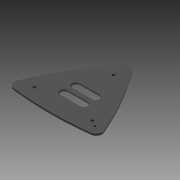
# Autodesk Inventor part: TOP PLATE
Saved by Autodesk Inventor 2013 (Build 170138000, 138)
## iProperties
Created: 2013-12-04
Part Number: TOP PLATE
Material: Generic
Document SubType Name: Modeling
Designer: employee
Density: 1 g/cm^3
Author: employee
Autodesk Inventor part; units mm, degrees
ref_plane "YZ Plane" through (0, 0, 0) normal (1, 0, 0) x (0, 1, 0)
ref_plane "XZ Plane" through (0, 0, 0) normal (0, 1, 0) x (-1, 0, 0)
ref_plane "XY Plane" through (0, 0, 0) normal (0, 0, 1) x (1, 0, 0)
sketch "Sketch1" plane through (0, 0, 0) normal (0, 0, 1) x (1, 0, 0)
  line L0 (0, -144.337567) -> (-125, 72.168784) construction
  line L1 (-125, 72.168784) -> (125, 72.168784) construction
  line L2 (125, 72.168784) -> (0, -144.337567) construction
  line L3 (0, 173.205081) -> (150, -86.60254) construction
  line L4 (150, -86.60254) -> (-150, -86.60254) construction
  line L5 (-150, -86.60254) -> (0, 173.205081) construction
  circle A0 centre (-150, -86.60254) radius 1.5875
  circle A1 centre (150, -86.60254) radius 1.5875
  circle A2 centre (0, 173.205081) radius 1.5875
  circle A3 centre (-125, 72.168784) radius 4.25
  circle A4 centre (125, 72.168784) radius 4.25
  circle A5 centre (0, -144.337567) radius 4.25
  circle A6 centre (-150, -86.60254) radius 25 construction
  line L6 (-250.015109, -144.34629) -> (0, 288.692581) construction
  line L7 (0, 288.692581) -> (250.015109, -144.34629) construction
  line L8 (250.015109, -144.34629) -> (-250.015109, -144.34629) construction
  arc A7 (-225.583531, -102.508939) -> (-201.567111, -144.106599) centre (-197.772126, -114.18379) ccw
  circle A8 centre (-125, 72.168784) radius 12.5 construction
  arc A9 (24.01642, 246.615539) -> (-24.01642, 246.615539) centre (0, 228.367581) ccw
  arc A10 (201.567111, -144.106599) -> (225.583531, -102.508939) centre (197.772126, -114.18379) ccw
  arc A11 (-24.01642, 246.615539) -> (-225.583531, -102.508939) centre (1251.593518, -722.607855) ccw
  arc A12 (225.583531, -102.508939) -> (24.01642, 246.615539) centre (-1251.593518, -722.607855) ccw
  arc A13 (-201.567111, -144.106599) -> (201.567111, -144.106599) centre (0, 1445.215709) ccw
  circle A14 centre (0, 228.367581) radius 1.5875
  circle A15 centre (-197.772126, -114.18379) radius 1.5875
  circle A16 centre (197.772126, -114.18379) radius 1.5875
  point P0 (0, 0)
  point P1 (0, 0)
  point P2 (0, 0)
  point P3 (0, 0)
  dimension "d0" = 300
  dimension "d1" = 250
  dimension "d2" = 3.175
  dimension "d3" = 8.5
  dimension "d4" = 50
  dimension "d5" = 60.325
  dimension "d6" = 25
  dimension "d9" = 3.175
  constraints: 18 end point, 17 centre point, 14 coincident, 14 tangent, 12 point on circle, 10 equal radius, 3 horizontal, 21 other
  measures "d0" distance of L3.end L4.end
  measures "d1" distance of L0.end L1.end
  measures "d2" diameter of A0
  measures "d3" diameter of A5
  measures "d4" diameter of A6
  measures "d5" diameter of A7
  measures "d6" diameter of A8
  measures "d9" diameter of A15
sketch "Sketch1 outline for Extrusion2" plane through (0, 0, 0) normal (0, 0, 1) x (1, 0, 0)
  arc A0 (-24.01642, 246.615539) -> (24.01642, 246.615539) centre (0, 228.367581) cw
  arc A1 (-225.583531, -102.508939) -> (-24.01642, 246.615539) centre (1251.593518, -722.607855) cw
  arc A2 (24.01642, 246.615539) -> (225.583531, -102.508939) centre (-1251.593518, -722.607855) cw
  arc A3 (-201.567111, -144.106599) -> (-225.583531, -102.508939) centre (-197.772126, -114.18379) cw
  arc A4 (225.583531, -102.508939) -> (201.567111, -144.106599) centre (197.772126, -114.18379) cw
  arc A5 (201.567111, -144.106599) -> (-201.567111, -144.106599) centre (0, 1445.215709) cw
  circle A6 centre (-197.772126, -114.18379) radius 1.5875
  circle A7 centre (-150, -86.60254) radius 1.5875
  circle A8 centre (197.772126, -114.18379) radius 1.5875
  circle A9 centre (150, -86.60254) radius 1.5875
  circle A10 centre (0, 228.367581) radius 1.5875
  circle A11 centre (0, 173.205081) radius 1.5875
extrude "Extrusion2" add sketch "Sketch1 outline for Extrusion2" along normal blind 12.5
sketch "Sketch8" plane through (0, 0, 0) normal (0, 0, -1) x (-1, 0, 0)
  circle A0 centre (0, 173.205081) radius 1.5875
  circle A1 centre (0, 173.205081) radius 11.5
  point P0 (0, 0)
  dimension "d34" = 23
  constraints: 1 centre point, 1 coincident
  measures "d34" diameter of A1
sketch "Sketch8 outline for Extrusion9" plane through (0, 0, 0) normal (0, 0, -1) x (-1, 0, 0)
  circle A0 centre (0, 173.205081) radius 11.5
  circle A1 centre (0, 173.205081) radius 1.5875
extrude "Extrusion9" cut sketch "Sketch8 outline for Extrusion9" against normal blind 7.9375
sketch "Sketch9" plane through (0, 173.205081, 7.9375) normal (0, 0, -1) x (-1, 0, 0)
  circle A0 centre (0, 0) radius 1.5875 projected
  circle A1 centre (0, 0) radius 11.5 projected
  circle A2 centre (0, 0) radius 7.5
  point P0 (0, -173.205081)
  dimension "d39" = 15
  constraints: 1 centre point, 1 coincident
  measures "d39" diameter of A2
sketch "Sketch9 outline for Extrusion10" plane through (0, 173.205081, 7.9375) normal (0, 0, -1) x (-1, 0, 0)
  circle A0 centre (0, 0) radius 7.5
  circle A1 centre (0, 0) radius 1.5875
extrude "Extrusion10" cut sketch "Sketch9 outline for Extrusion10" against normal through all
pattern_circular "Circular Pattern1" count 3 over 360 about axis through (0, 0, -10) along (0, 0, 1) of "Extrusion9", "Extrusion10"
sketch "Sketch10" plane through (0, 0, 0) normal (0, 0, -1) x (-1, 0, 0)
  line L0 (-50, 12.5) -> (50, 12.5)
  arc A0 (50, 12.5) -> (50, 50) centre (50, 31.25) ccw
  line L1 (50, 50) -> (-50, 50)
  arc A1 (-50, 50) -> (-50, 12.5) centre (-50, 31.25) ccw
  line L2 (-50, -12.5) -> (50, -12.5)
  arc A2 (50, -50) -> (50, -12.5) centre (50, -31.25) ccw
  line L3 (50, -50) -> (-50, -50)
  arc A3 (-50, -12.5) -> (-50, -50) centre (-50, -31.25) ccw
  line L4 (0, 0) -> (0, -12.5)
  line L5 (0, 0) -> (0, 12.5)
  dimension "d46" = 25
  dimension "d48" = 100
  dimension "d49" = 18.75
  constraints: 12 end point, 8 point on circle, 8 tangent, 4 centre point, 4 equal length, 3 vertical alignment, 2 midpoint, 1 collinear, 1 equal radius, 1 horizontal
  measures "d46" distance between parallel lines of L0 L2
  measures "d48" distance of L2.start L2.end
  measures "d49" radius of A2
sketch "Sketch10 outline for Extrusion11" plane through (0, 0, 0) normal (0, 0, -1) x (-1, 0, 0)
  line L0 (50, -12.5) -> (-50, -12.5)
  arc A0 (-50, -12.5) -> (-50, -50) centre (-50, -31.25) ccw
  line L1 (-50, -50) -> (50, -50)
  arc A1 (50, -50) -> (50, -12.5) centre (50, -31.25) ccw
  line L2 (-50, 12.5) -> (50, 12.5)
  arc A2 (50, 12.5) -> (50, 50) centre (50, 31.25) ccw
  line L3 (50, 50) -> (-50, 50)
  arc A3 (-50, 50) -> (-50, 12.5) centre (-50, 31.25) ccw
extrude "Extrusion11" cut sketch "Sketch10 outline for Extrusion11" against normal through all
sketch "Sketch11" plane through (0, 0, 0) normal (0, 0, -1) x (-1, 0, 0)
  circle A0 centre (-150, -86.60254) radius 11.5
  arc A1 (-225.583531, -102.508939) -> (-201.567111, -144.106599) centre (-197.772126, -114.18379) ccw
  circle A2 centre (-197.772126, -114.18379) radius 12.5
  circle A3 centre (-197.772126, -114.18379) radius 25
  circle A4 centre (-181.53415, -104.80879) radius 6.25
  line L0 (-197.772126, -114.18379) -> (-181.53415, -104.80879)
  line L1 (-150, -86.60254) -> (-181.53415, -104.80879)
  point P0 (0, 0)
  dimension "d52" = 25
  dimension "d54" = 50
  constraints: 4 end point, 3 centre point, 2 coincident, 2 tangent, 1 collinear
  measures "d52" diameter of A2
  measures "d54" diameter of A3
sketch "Sketch11 outline for Extrusion12" plane through (0, 0, 0) normal (0, 0, -1) x (-1, 0, 0)
  circle A0 centre (-181.53415, -104.80879) radius 6.25
extrude "Extrusion12" cut sketch "Sketch11 outline for Extrusion12" against normal through all
fillet "Fillet2" radius 6.35 22 edges at (-68.75, 31.25, 0) (0, 12.5, 0) (68.75, 31.25, 0) (0, 50, 0) (68.75, 31.25, 12.5) (0, 12.5, 12.5) (-68.75, 31.25, 12.5) (0, 50, 12.5) (-68.75, -31.25, 0) (0, -50, 0) (68.75, -31.25, 0) (0, -12.5, 0) (68.75, -31.25, 12.5) (0, -50, 12.5) (-68.75, -31.25, 12.5) (0, -12.5, 12.5) (223.8936, -129.265, 0) (0, -156.8376, 0) (-223.8936, -129.265, 0) (-135.8253, 78.4188, 0) (0, 258.5301, 0) (135.8253, 78.4188, 0)
body "Solid2"
